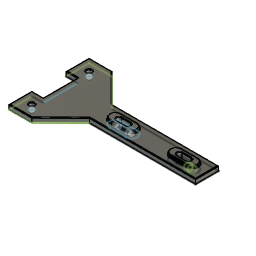
Soporte PSU v1 (Autodesk Fusion 360 design; units mm, degrees)
Autodesk Fusion 360 part; units mm, degrees
sketch "Boceto1" plane through (0, 0, 0) normal (0, 0, 1) x (1, 0, 0)
  line L0 (-50.0315, 50) -> (-50.0315, 70)
  line L1 (-50.0315, 50) -> (-40, 50)
  line L2 (-40, 50) -> (-40, 20)
  line L3 (-40, 20) -> (-50, 20)
  line L4 (-50, 20) -> (-50, 0)
  line L5 (-50, 0) -> (-30, 0)
  line L6 (-30, 0) -> (-4.6279, 25)
  line L7 (-4.6279, 25) -> (88, 25)
  line L8 (88, 25) -> (88, 45)
  line L9 (88, 45) -> (-5, 45)
  line L10 (-5, 45) -> (-30.0315, 70)
  line L11 (-30.0315, 70) -> (-50.0315, 70)
  line L12 (72, 37.1) -> (64, 37.1)
  arc A0 (64, 37.1) -> (64, 32.9) centre (64, 35) ccw
  line L13 (64, 32.9) -> (72, 32.9)
  arc A1 (72, 32.9) -> (72, 37.1) centre (72, 35) ccw
  line L14 (19, 37.1) -> (11, 37.1)
  arc A2 (11, 37.1) -> (11, 32.9) centre (11, 35) ccw
  line L15 (11, 32.9) -> (19, 32.9)
  arc A3 (19, 32.9) -> (19, 37.1) centre (19, 35) ccw
  arc A4 (8, 40) -> (8, 30) centre (8, 35) ccw
  line L16 (8, 30) -> (22, 30)
  arc A5 (22, 30) -> (22, 40) centre (22, 35) ccw
  line L17 (22, 40) -> (8, 40)
  arc A6 (61, 40) -> (61, 30) centre (61, 35) ccw
  line L18 (61, 30) -> (75, 30)
  arc A7 (75, 30) -> (75, 40) centre (75, 35) ccw
  line L19 (75, 40) -> (61, 40)
  circle A8 centre (-40.0315, 60) radius 2.1
  circle A9 centre (-40, 10) radius 2.1
  dimension "d1" = 20
  dimension "d4" = 30
  dimension "d5" = 20
  dimension "d6" = 20
  dimension "d7" = 20
  dimension "d8" = 20
  dimension "d10" = 8
  dimension "d11" = 4.2
  dimension "d12" = 16
  dimension "d13" = 7.9
  dimension "d14" = 8
  dimension "d15" = 4.2
  dimension "d16" = 45
  dimension "d17" = 14
  dimension "d18" = 10
  dimension "d19" = 3
  dimension "d20" = 14
  dimension "d21" = 10
  dimension "d22" = 3
  dimension "d23" = 4.2
  dimension "d24" = 4.2
  constraint vertical L0
  constraint perpendicular L0 L1
  constraint perpendicular L1 L2
  constraint perpendicular L2 L3
  constraint perpendicular L3 L4
  constraint perpendicular L4 L5
  constraint perpendicular L2 L7
  constraint perpendicular L5 L8
  constraint perpendicular L8 L9
  constraint perpendicular L0 L11
  constraint horizontal L12
  constraint tangent L12 A0
  constraint tangent A0 L13
  constraint parallel L12 L13
  constraint tangent L13 A1
  constraint tangent L12 A1
  constraint horizontal L14
  constraint tangent L14 A2
  constraint tangent A2 L15
  constraint parallel L14 L15
  constraint tangent L15 A3
  constraint tangent L14 A3
  constraint horizontal L17
  constraint tangent A4 L17
  constraint tangent A4 L16
  constraint parallel L16 L17
  constraint tangent L16 A5
  constraint tangent A5 L17
  constraint horizontal L19
  constraint tangent A6 L19
  constraint tangent A6 L18
  constraint parallel L18 L19
  constraint tangent L18 A7
  constraint tangent A7 L19
  measures "d1" distance of L0.start L0.end
  measures "d4" distance of L1.end L2.end
  measures "d5" distance of L3.end L4.end
  measures "d6" distance of L7.end L8.end
  measures "d7" distance of L0.end L10.end
  measures "d8" distance of L4.end L5.end
  measures "d10" distance of L12.start L12.end
  measures "d11" distance of L12.end A0.end
  measures "d12" horizontal distance of L8.end A1.centre
  measures "d13" distance of L9 L12.start
  measures "d14" distance of L14.start L14.end
  measures "d15" distance of A2.end L14.end
  measures "d16" distance of A0.centre A3.centre
  measures "d17" distance of A4.start A5.end
  measures "d18" distance of A4.end A4.start
  measures "d19" distance of A2.centre A4.centre
  measures "d20" distance of A6.start A7.end
  measures "d21" distance of A6.start A6.end
  measures "d22" distance of A0.centre A6.centre
  measures "d23" diameter of A8
  measures "d24" diameter of A9
extrude "Extruir1" add sketch "Boceto1" along normal blind 6 contours A4 L16 A5 L17 | A6 L18 A7 L19 makes body 1 at (13.6667, 39.0333, 0) makes body 2 at (69.3333, 30.9667, 0)
extrude "Extruir2" add sketch "Boceto1" along normal blind 4 contours L0 L1 L2 L3 L4 L5 L6 L7 L8 L9 L10 L11 bodies 1 2
fillet "Empalme1" radius 0.5 11 faces at (-28.3333, 38.3333, 4) (13.6667, 39.0333, 6) (69.3333, 30.9667, 6) (3.4425, 32.9436, 4.6667) (12.6667, 30, 4.6667) (23.9422, 39.6074, 4.6667) (17.3333, 40, 4.6667) (59.7662, 39.8454, 5.3333) (65.6667, 30, 4.6667) (76.9422, 39.6074, 4.6667) (70.3333, 40, 4.6667) on bodies 1
